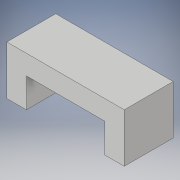
# Autodesk Inventor part: Cpiece
Saved by Autodesk Inventor 2019 (Build 230136000, 136)
## iProperties
Created: 2019-10-26
Part Number: Cpiece
Material: Generic
Document SubType Name: Modeling
Designer: test
Density: 1 g/cm^3
Appearance: Default
Author: test
Autodesk Inventor part; units mm, degrees
ref_plane "YZ Plane" through (0, 0, 0) normal (1, 0, 0) x (0, 1, 0)
ref_plane "XZ Plane" through (0, 0, 0) normal (0, 1, 0) x (-1, 0, 0)
ref_plane "XY Plane" through (0, 0, 0) normal (0, 0, 1) x (1, 0, 0)
sketch "Sketch1" plane through (0, 0, 0) normal (0, 1, 0) x (-1, 0, 0)
  line L0 (-26.4284, 51.2097) -> (59.9316, 51.2097)
  line L1 (31.9916, 28.3497) -> (37.0716, 28.3497)
  line L2 (37.0716, 28.3497) -> (37.0716, 15.6497)
  line L3 (37.0716, 15.6497) -> (31.9916, 15.6497)
  line L4 (31.9916, 15.6497) -> (31.9916, 28.3497)
  line L5 (31.9916, 28.3497) -> (37.0716, 15.6497) construction
  line L6 (37.0716, 28.3497) -> (31.9916, 15.6497) construction
  line L7 (34.5316, 51.2097) -> (34.5316, -7.2103) construction
  line L8 (59.9316, -7.2103) -> (-26.4284, -7.2103) construction
  line L9 (9.1316, 51.2097) -> (9.1316, -7.2103) construction
  line L10 (6.5916, 28.3497) -> (11.6716, 28.3497)
  line L11 (11.6716, 28.3497) -> (11.6716, 15.6497)
  line L12 (11.6716, 15.6497) -> (6.5916, 15.6497)
  line L13 (6.5916, 15.6497) -> (6.5916, 28.3497)
  line L14 (6.5916, 28.3497) -> (11.6716, 15.6497) construction
  line L15 (11.6716, 28.3497) -> (6.5916, 15.6497) construction
  point P0 (0, 0)
  point P1 (34.5316, 21.9997)
  point P2 (34.5316, 21.9997)
  point P3 (9.1316, 21.9997)
  point P4 (9.1316, 21.9997)
  dimension "d4" = 12.7
  dimension "d5" = 5.08
  dimension "d7" = 25.4
  constraints: 32 end point, 6 midpoint, 2 horizontal, 2 parallel, 1 perpendicular, 1 point on line, 1 vertical, 15 other
  measures "d4" distance of L1.end L2.end
  measures "d5" distance of L2.end L3.end
  measures "d7" distance of L7.start L9.start
extrude "Extrusion1" add sketch "Sketch1" along normal blind 7.62
sketch "Sketch3" plane through (0, 7.62, 0) normal (0, 1, 0) x (1, 0, 0)
  line L0 (-37.0716, -15.6497) -> (-37.0716, -28.3497) projected
  line L1 (-6.5916, -15.6497) -> (-6.5916, -28.3497) projected
  line L2 (-37.0716, -15.6497) -> (-6.5916, -15.6497)
  line L3 (-6.5916, -15.6497) -> (-6.5916, -28.3497)
  line L4 (-6.5916, -28.3497) -> (-37.0716, -28.3497)
  line L5 (-37.0716, -28.3497) -> (-37.0716, -15.6497)
  point P0 (0, 0)
  constraints: 8 end point, 2 parallel, 1 horizontal, 1 perpendicular
extrude "Extrusion2" add sketch "Sketch3" along normal blind 5.08
body "Solid1"
